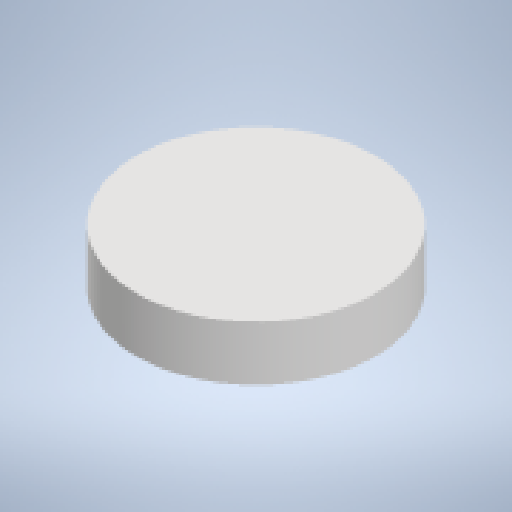
# Autodesk Inventor part: stock material 1
Saved by Autodesk Inventor 2023.2 (Build 272271030, 271C)
## iProperties
Created: 2023-07-31
Part Number: stock material 1
Material: Generic
Document SubType Name: Modeling
Designer: Cris Pat
Density: 1 g/cm^3
Appearance: Default
Author: Cris Pat
Autodesk Inventor part; units mm, degrees
ref_plane "YZ Plane" through (0, 0, 0) normal (1, 0, 0) x (0, 1, 0)
ref_plane "XZ Plane" through (0, 0, 0) normal (0, 1, 0) x (-1, 0, 0)
sketch "Sketch1" plane through (0, 0, 0) normal (0, 0, 1) x (1, 0, 0)
  line L0 (0, 0) -> (0, 76.2) construction
  line L1 (76.2, 0) -> (0, 0) construction
  line L2 (76.2, 76.2) -> (76.2, 0) construction
  line L3 (0, 76.2) -> (76.2, 76.2) construction
  circle A0 centre (38.1, 38.1) radius 35.1
  dimension "d0" = 38.1
  dimension "d1" = 38.1
  dimension "d2" = 3
  constraints: 1 centre point
  measures "d0" horizontal distance of L0.start A0.centre
  measures "d1" horizontal distance of L0.start A0.centre
  measures "d2" distance edge to line of A0 L3
ref_plane "Work Plane1" through (-3.81, -3.81, -16.05) normal (0, 0, 1) x (1, 0, 0)
extrude "Extrusion1" add sketch "Sketch1" against normal up to surface (16.05 mm away)
body "Solid1"
